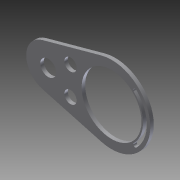
# Autodesk Inventor part: back plate
Saved by Autodesk Inventor 2012 (Build 160160000, 160)
## iProperties
Created: 2012-01-30
Part Number: back plate
Material: Default
Document SubType Name: Modeling
Designer: Antonella Wilby
Density: 1 g/cm^3
Author: Antonella Wilby
Autodesk Inventor part; units mm, degrees
ref_plane "YZ Plane" through (0, 0, 0) normal (1, 0, 0) x (0, 1, 0)
ref_plane "XZ Plane" through (0, 0, 0) normal (0, 1, 0) x (-1, 0, 0)
ref_plane "XY Plane" through (0, 0, 0) normal (0, 0, 1) x (1, 0, 0)
sketch "Sketch1" plane through (0, 0, 0) normal (0, 0, 1) x (1, 0, 0)
  line L0 (-198.755, 0) -> (114.6175, 0) projected
  line L1 (0, -97.79) -> (0, 97.79) projected
  circle A0 centre (0, 0) radius 50.8 construction
  arc A1 (-18.4326, -67.374) -> (-18.4326, 67.374) centre (0, 0) ccw
  arc A2 (44.9013, -44.9013) -> (44.9013, 44.9013) centre (0, 0) ccw
  arc A3 (40.1305, -40.1305) -> (40.1305, 40.1305) centre (0, 0) ccw
  line L2 (0, 0) -> (44.9013, 44.9013) construction
  line L3 (0, 0) -> (44.9013, -44.9013) construction
  arc A4 (44.9013, 44.9013) -> (40.1305, 40.1305) centre (42.5159, 42.5159) ccw
  arc A5 (40.1305, -40.1305) -> (44.9013, -44.9013) centre (42.5159, -42.5159) ccw
  circle A6 centre (-114.3, 0) radius 14.2875
  arc A7 (-124.7731, 38.2807) -> (-124.7731, -38.2807) centre (-114.3, 0) ccw
  line L4 (-114.3, -14.2875) -> (-114.3, 14.2875) construction
  line L5 (-124.7731, 38.2807) -> (-18.4326, 67.374)
  line L6 (-124.7731, -38.2807) -> (-18.4326, -67.374)
  circle A8 centre (-74.0404, 25.4) radius 11.1125
  circle A9 centre (-74.0404, -25.4) radius 11.1125
  circle A10 centre (0, 0) radius 19.05
  circle A11 centre (0, 0) radius 53.975
  dimension "d0" = 101.6
  dimension "d1" = 19.05
  dimension "d2" = 6.7469
  dimension "d3" = 6.35
  dimension "d6" = 28.575
  dimension "d7" = 25.4
  dimension "d9" = 22.225
  dimension "d10" = 38.1
  dimension "d11" = 45
  dimension "d12" = 45
  dimension "d13" = 3.175
  dimension "d14" = 114.3
  constraints: 14 point on circle, 12 centre point, 10 end point, 6 coincident, 6 tangent, 2 horizontal alignment, 2 midpoint, 2 point on line, 1 parallel
  measures "d0" diameter of A0
  measures "d1" radial gap between concentric circles of A1 A0
  measures "d2" radial gap between concentric circles of A2 A3
  measures "d3" radial gap between concentric circles of A1 A2
  measures "d6" diameter of A6
  measures "d7" radial gap between concentric circles of A7 A6
  measures "d9" diameter of A8
  measures "d10" diameter of A10
  measures "d11" angle of L0 L3
  measures "d12" angle of L2 L0
  measures "d13" radial gap between concentric circles of A11 A0
  measures "d14" distance between parallel lines of L1 L4
extrude "Extrusion1" add sketch "Sketch1" along normal mid plane 6.35 contours A11 L1 A1 L0 A2 A4 A3 | L0 A3 A5 A2 A1 L1 A11 | A11 L0 A6 A7 L5 A1 L1 | L1 A1 L6 A7 L0 A6 A11
body "Solid1"
